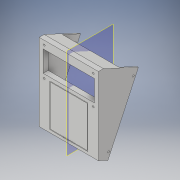
# Autodesk Inventor part: face
Saved by Autodesk Inventor 2017 (Build 210142000, 142)
## iProperties
Created: 2018-01-22
Part Number: face
Material: Generic
Document SubType Name: Modeling
Designer: chuck
Density: 1 g/cm^3
Appearance: Default
Author: chuck
Autodesk Inventor part; units mm, degrees
ref_plane "YZ Plane" through (0, 0, 0) normal (1, 0, 0) x (0, 1, 0)
ref_plane "XZ Plane" through (0, 0, 0) normal (0, 1, 0) x (-1, 0, 0)
ref_plane "XY Plane" through (0, 0, 0) normal (0, 0, 1) x (1, 0, 0)
sketch "Sketch1" plane through (0, 0, 0) normal (0, 0, 1) x (1, 0, 0)
  line L0 (0, 0) -> (112.522, 0)
  line L1 (112.522, 0) -> (112.522, 146.812)
  line L2 (112.522, 146.812) -> (0, 146.812)
  line L3 (0, 146.812) -> (0, 0)
  line L4 (7.62, 131.572) -> (104.902, 131.572)
  line L5 (104.902, 131.572) -> (104.902, 91.44)
  line L6 (104.902, 91.44) -> (7.62, 91.44)
  line L7 (7.62, 91.44) -> (7.62, 131.572)
  line L8 (21.59, 83.82) -> (90.932, 83.82)
  line L9 (90.932, 83.82) -> (90.932, 6.35)
  line L10 (90.932, 6.35) -> (21.59, 6.35)
  line L11 (21.59, 6.35) -> (21.59, 83.82)
  dimension "d0" = 97.282
  dimension "d1" = 40.132
  dimension "d2" = 69.342
  dimension "d3" = 77.47
  dimension "d4" = 6.35
  dimension "d5" = 21.59
  dimension "d6" = 7.62
  dimension "d7" = 7.62
  dimension "d8" = 15.24
  dimension "d9" = 7.62
  constraints: 24 end point, 6 parallel, 3 horizontal, 3 perpendicular
  measures "d0" distance of L4.start L4.end
  measures "d1" distance of L6.end L4.start
  measures "d2" distance of L8.start L8.end
  measures "d3" distance of L10.end L8.start
  measures "d4" distance between parallel lines of L0 L10
  measures "d5" distance between parallel lines of L3 L11
  measures "d6" distance between parallel lines of L3 L7
  measures "d7" distance between parallel lines of L1 L5
  measures "d8" distance between parallel lines of L2 L4
  measures "d9" distance between parallel lines of L6 L8
extrude "Extrusion1" add sketch "Sketch1" along normal blind 9.4996 contours L3 L2 L1 L0 | L8 L9 L10 L11
sketch "Sketch2" plane through (0, 0, 9.4996) normal (0, 0, 1) x (1, 0, 0)
  line L0 (0, 0) -> (112.522, 0)
  line L1 (112.522, 0) -> (112.522, 139.192)
  line L2 (112.522, 139.192) -> (0, 139.192)
  line L3 (0, 139.192) -> (0, 0)
  line L4 (7.62, 131.572) -> (104.902, 131.572)
  line L5 (104.902, 131.572) -> (104.902, 91.44)
  line L6 (104.902, 91.44) -> (7.62, 91.44)
  line L7 (7.62, 91.44) -> (7.62, 131.572)
  line L8 (21.59, 83.82) -> (90.932, 83.82)
  line L9 (90.932, 83.82) -> (90.932, 6.35)
  line L10 (90.932, 6.35) -> (21.59, 6.35)
  line L11 (21.59, 6.35) -> (21.59, 83.82)
  line L12 (20.32, 85.09) -> (92.202, 85.09)
  line L13 (92.202, 85.09) -> (92.202, 5.08)
  line L14 (92.202, 5.08) -> (20.32, 5.08)
  line L15 (20.32, 5.08) -> (20.32, 85.09)
  dimension "d12" = 97.282
  dimension "d13" = 40.132
  dimension "d14" = 69.342
  dimension "d15" = 77.47
  dimension "d16" = 6.35
  dimension "d17" = 21.59
  dimension "d18" = 7.62
  dimension "d19" = 7.62
  dimension "d20" = 7.62
  dimension "d21" = 7.62
  dimension "d33" = 1.27
  dimension "d34" = 1.27
  dimension "d35" = 1.27
  dimension "d36" = 1.27
  constraints: 32 end point, 8 parallel, 4 horizontal, 4 perpendicular
  measures "d12" distance of L4.start L4.end
  measures "d13" distance of L6.end L4.start
  measures "d14" distance of L8.start L8.end
  measures "d15" distance of L10.end L8.start
  measures "d16" distance between parallel lines of L0 L10
  measures "d17" distance between parallel lines of L3 L11
  measures "d18" distance between parallel lines of L3 L7
  measures "d19" distance between parallel lines of L1 L5
  measures "d20" distance between parallel lines of L2 L4
  measures "d21" distance between parallel lines of L6 L8
  measures "d33" distance between parallel lines of L13 L9
  measures "d34" distance between parallel lines of L12 L8
  measures "d35" distance between parallel lines of L15 L11
  measures "d36" distance between parallel lines of L10 L14
extrude "Extrusion2" cut sketch "Sketch2" against normal blind 0.0025 contours L12 L13 L14 L15
sketch "Sketch3" plane through (0, 0, 9.4996) normal (0, 0, 1) x (1, 0, 0)
  circle A0 centre (9.7155, 138.9888) radius 1.651
  circle A1 centre (102.7811, 138.9888) radius 1.651
  circle A2 centre (102.7811, 84.0232) radius 1.651
  circle A3 centre (9.7155, 84.0232) radius 1.651
  line L0 (104.902, 131.572) -> (104.902, 91.44) projected
  line L1 (104.902, 91.44) -> (7.62, 91.44) projected
  line L2 (21.59, 6.35) -> (90.932, 6.35) projected
  line L3 (92.202, 5.08) -> (20.32, 5.08) projected
  line L4 (46.101, 6.35) -> (66.421, 6.35)
  line L5 (66.421, 6.35) -> (66.421, 5.08)
  line L6 (66.421, 5.08) -> (46.101, 5.08)
  line L7 (46.101, 5.08) -> (46.101, 6.35)
  line L8 (21.59, 83.82) -> (21.59, 6.35) projected
  line L9 (90.932, 6.35) -> (90.932, 83.82) projected
  point P0 (0, 0)
  dimension "d24" = 3.302
  dimension "d25" = 93.0656
  dimension "d26" = 93.0656
  dimension "d27" = 0
  dimension "d28" = 54.9656
  dimension "d29" = 2.1209
  dimension "d30" = 0
  dimension "d31" = 7.4168
  dimension "d32" = 0
  dimension "d37" = 20.32
  dimension "d38" = 24.511
  dimension "d39" = 24.511
  constraints: 8 end point, 4 centre point, 3 equal radius, 2 parallel, 2 point on line, 1 horizontal, 1 perpendicular
  measures "d24" diameter of A1
  measures "d25" distance of A1.centre A0.centre
  measures "d26" distance of A2.centre A3.centre
  measures "d27" vertical distance of A2.centre A3.centre
  measures "d28" distance of A0.centre A3.centre
  measures "d29" distance from line of L0 A1.centre
  measures "d30" vertical distance of A1.centre A0.centre
  measures "d31" distance from line of L1 A2.centre
  measures "d32" horizontal distance of A0.centre A3.centre
  measures "d37" distance between parallel lines of L5 L7
  measures "d38" distance between parallel lines of L8 L7
  measures "d39" distance between parallel lines of L9 L5
extrude "Extrusion3" cut sketch "Sketch3" against normal through all
sketch "Sketch10" plane through (0, 0, 0) normal (0, 0, -1) x (-1, 0, 0)
  line L0 (12.7738, 184.0109) -> (-117.8029, 184.0109)
  line L1 (-117.8029, 184.0109) -> (-117.8029, -18.4511)
  line L2 (-117.8029, -18.4511) -> (12.7738, -18.4511)
  line L3 (12.7738, -18.4511) -> (12.7738, 184.0109)
  line L4 (-5.08, 138.9888) -> (-5.08, 84.0232)
  line L5 (-14.351, 134.112) -> (-98.1202, 134.112)
  line L6 (-107.442, 138.9888) -> (-107.442, 84.0232)
  line L7 (-112.522, 0) -> (-112.522, 146.812) projected
  line L8 (-14.351, 88.9) -> (-98.1202, 88.9)
  arc A0 (-5.08, 138.9888) -> (-14.351, 138.9888) centre (-9.7155, 138.9888) ccw
  arc A1 (-14.351, 84.0232) -> (-5.08, 84.0232) centre (-9.7155, 84.0232) ccw
  arc A2 (-107.442, 84.0232) -> (-98.1202, 84.0232) centre (-102.7811, 84.0232) ccw
  arc A3 (-98.1202, 138.9888) -> (-107.442, 138.9888) centre (-102.7811, 138.9888) ccw
  circle A4 centre (-9.7155, 84.0232) radius 1.651 projected
  circle A5 centre (-9.7155, 138.9888) radius 1.651 projected
  circle A6 centre (-102.7811, 138.9888) radius 1.651 projected
  circle A7 centre (-102.7811, 84.0232) radius 1.651 projected
  line L9 (-14.351, 134.112) -> (-14.351, 138.9888)
  line L10 (-98.1202, 138.9888) -> (-98.1202, 134.112)
  line L11 (-7.62, 131.572) -> (-7.62, 91.44) projected
  line L12 (-7.62, 131.572) -> (-104.902, 131.572) projected
  line L13 (-7.62, 91.44) -> (-104.902, 91.44) projected
  line L14 (-104.902, 131.572) -> (-104.902, 91.44) projected
  line L15 (-98.1202, 84.0232) -> (-98.1202, 88.9)
  line L16 (-14.351, 88.9) -> (-14.351, 84.0232)
  line L17 (0, 76.2) -> (-112.5015, 3.0431)
  line L18 (-112.5015, 3.0431) -> (-112.522, 0)
  line L19 (-112.522, 0) -> (1.3847, 74.0706)
  line L20 (1.3847, 74.0706) -> (0, 76.2)
  line L21 (1.524, 2.54) -> (-112.522, 76.2)
  line L22 (-112.522, 76.2) -> (-114.4017, 74.3903)
  line L23 (-114.4017, 74.3903) -> (0.1459, 0.4063)
  line L24 (0.1459, 0.4063) -> (1.524, 2.54)
  line L25 (0, 0) -> (-112.522, 0) projected
  line L26 (0, 146.812) -> (0, 0) projected
  point P0 (-14.351, 136.5504)
  dimension "d64" = 2.54
  dimension "d65" = 2.54
  dimension "d66" = 2.54
  dimension "d67" = 2.54
  dimension "d68" = 2.54
  dimension "d69" = 2.54
  dimension "d70" = 2.54
  dimension "d71" = 1.524
  dimension "d72" = 76.2
  dimension "d73" = 0
  dimension "d74" = 76.2
  dimension "d75" = 0
  dimension "d76" = 0
  dimension "d77" = 0
  constraints: 40 end point, 8 point on circle, 8 tangent, 6 parallel, 4 centre point, 4 concentric, 4 vertical, 3 horizontal, 3 perpendicular, 1 midpoint
  measures "d64" distance between parallel lines of L11 L4
  measures "d65" distance between parallel lines of L12 L5
  measures "d66" distance between parallel lines of L13 L8
  measures "d67" distance between parallel lines of L14 L6
  measures "d68" distance between parallel lines of L19 L17
  measures "d69" distance between parallel lines of L21 L23
  measures "d70" vertical distance of L25.start L21.start
  measures "d71" horizontal distance of L25.start L21.start
  measures "d72" distance from line of L25 L17.start
  measures "d73" distance from line of L26 L17.start
  measures "d74" distance from line of L25 L21.end
  measures "d75" distance from line of L7 L21.end
  measures "d76" distance from line of L25 L18.end
  measures "d77" distance from line of L7 L18.end
extrude "Extrusion8" cut sketch "Sketch10" against normal blind 6.858 contours L3 L2 L1 L0 | L7 L23 L17 L18 | L19 L23 L26 L25 | L19 L26 L21
sketch "Sketch5" plane through (112.522, 0, 9.4996) normal (1, 0, 0) x (0, 0, -1)
  line L0 (9.4996, 146.812) -> (0, 146.812) projected
  line L1 (9.4996, 146.812) -> (75.9867, 115.8086)
  line L2 (9.4996, 0) -> (0, 0) projected
  line L3 (18.0577, -8.4205) -> (0, 0)
  line L4 (0, 146.812) -> (0, 0) projected
  line L5 (0, 0) -> (0, 146.812)
  line L6 (0, 146.812) -> (9.4996, 146.812)
  line L7 (75.9867, 115.8086) -> (18.0577, -8.4205)
  line L8 (22.86, 146.812) -> (22.86, 73.406)
  line L9 (9.4996, 0) -> (9.4996, 146.812) projected
  point P0 (5.08, 0)
  point P1 (9.4996, 80.01)
  point P2 (22.86, 80.01)
  dimension "d45" = 25
  dimension "d47" = 22.86
  dimension "d48" = 33.02
  constraints: 12 end point, 2 perpendicular, 1 collinear, 1 parallel, 1 point on line, 1 vertical
  measures "d45" angle of L0 L1
  measures "d47" distance between parallel lines of L8 L4
  measures "d48" distance from line of point (22.86, 80.01) L7
extrude "Extrusion5" add sketch "Sketch5" against normal blind 2.54
ref_plane "Work Plane1" through (56.261, 0, 9.4996) normal (-1, 0, 0) x (0, 0, 1)
mirror "Mirror1" about plane through (56.261, 0, 9.4996) normal (-1, 0, 0) of "Extrusion5"
sketch "Sketch7" plane through (112.522, 0, 9.4996) normal (1, 0, 0) x (0, 0, -1)
  line L0 (18.0577, -8.4205) -> (0, 0) projected
  line L1 (0, 0) -> (18.0577, -8.4205)
  line L2 (18.0577, -8.4205) -> (19.1312, -6.1184)
  line L3 (75.9867, 115.8086) -> (18.0577, -8.4205) projected
  line L4 (0, 2.8026) -> (0, 0)
  line L5 (0.0025, 6.35) -> (0.0025, 83.82) projected
  line L6 (19.1312, -6.1184) -> (0, 2.8026)
  line L7 (9.4996, 146.812) -> (0, 146.812) projected
  line L8 (9.4996, 146.812) -> (9.4996, 144.0094)
  line L9 (9.4996, 146.812) -> (9.4996, 0) projected
  line L10 (9.4996, 144.0094) -> (40.3829, 129.6083)
  line L11 (40.3829, 129.6083) -> (41.4564, 131.9103)
  line L12 (9.4996, 146.812) -> (75.9867, 115.8086) projected
  line L13 (41.4564, 131.9103) -> (9.4996, 146.812)
  line L14 (0, 146.812) -> (9.4996, 146.812)
  line L15 (9.4996, 144.0094) -> (0, 144.0094)
  line L16 (0, 146.812) -> (0, 0) projected
  line L17 (0, 144.0094) -> (0, 146.812)
  point P0 (9.4996, 80.01)
  point P1 (2.6416, 146.812)
  dimension "d51" = 2.54
  dimension "d61" = 2.54
  dimension "d63" = 38.1
  constraints: 22 end point, 5 point on line, 3 perpendicular, 2 collinear, 2 parallel
  measures "d51" distance between parallel lines of L6 L0
  measures "d61" distance between parallel lines of L12 L10
  measures "d63" distance from line of L3.start L11
extrude "Extrusion6" add sketch "Sketch7" against normal through all contours L0 L4 L6 L2 | L16 L7 L8 L15 | L11 L10 L8 L12
sketch "Sketch8" plane through (112.522, 0, 9.4996) normal (1, 0, 0) x (0, 0, -1)
  circle A0 centre (19.1087, 5.1024) radius 1.5875
  circle A1 centre (66.3031, 106.3112) radius 1.5875
  line L0 (0, 0) -> (18.0577, -8.4205) projected
  line L1 (18.0577, -8.4205) -> (75.9867, 115.8086) projected
  line L2 (75.9867, 115.8086) -> (9.4996, 146.812) projected
  point P0 (9.4996, 0)
  dimension "d54" = 3.175
  dimension "d55" = 12.7
  dimension "d56" = 4.7625
  dimension "d57" = 4.7625
  dimension "d80" = 12.7
  constraints: 2 centre point, 1 equal radius
  measures "d54" diameter of A0
  measures "d55" distance from line of A0.centre L0
  measures "d56" distance from line of A0.centre L1
  measures "d57" distance from line of L1 A1.centre
  measures "d80" distance from line of L2 A1.centre
extrude "Extrusion7" cut sketch "Sketch8" against normal through all
body "Solid1"
